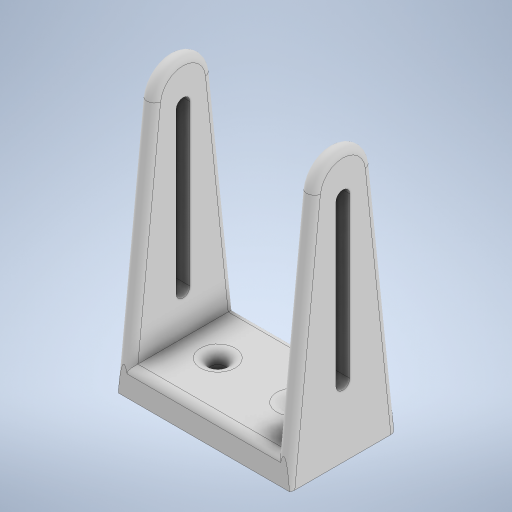
# Autodesk Inventor part: podstawa raspberry
Saved by Autodesk Inventor 2023 (Build 270158000, 158)
## iProperties
Created: 2023-04-25
Part Number: podstawa raspberry
Material: Ogólny
Document SubType Name: Modeling
Designer: janek
Density: 1 g/cm^3
Appearance: Domyślna
Author: janek
## iProperties of the stored document Zewnetrzny_stojak_Drukowanie 3D.ipt
Created: 2023-04-25
Part Number: Zewnetrzny_stojak_Drukowanie 3D
Material: Ogólny
Document SubType Name: Modeling
Designer: janek
Density: 1 g/cm^3
Appearance: Domyślna
Author: janek
Autodesk Inventor part; units mm, degrees
ref_plane "YZ Plane" through (0, 0, 0) normal (1, 0, 0) x (0, 1, 0)
ref_plane "XZ Plane" through (0, 0, 0) normal (0, 1, 0) x (-1, 0, 0)
ref_plane "XY Plane" through (0, 0, 0) normal (0, 0, 1) x (1, 0, 0)
sketch "Szkic1" plane through (0, 0, 0) normal (0, 1, 0) x (-1, 0, 0)
  line L0 (25.5952, -5.4437) -> (-24.4048, -5.4437)
  line L1 (-24.4048, -5.4437) -> (-24.4048, -35.4437)
  line L2 (-24.4048, -35.4437) -> (25.5952, -35.4437)
  line L3 (25.5952, -35.4437) -> (25.5952, -5.4437)
  point P0 (0, 0)
  point P1 (0.5952, -5.4437)
  point P2 (0.5952, -35.4437)
  dimension "d0" = 50
  dimension "d1" = 30
  constraints: 8 end point, 2 midpoint, 2 parallel, 1 horizontal, 1 perpendicular
  measures "d0" distance between parallel lines of L3 L1
  measures "d1" distance of point (0.595, -5.444) point (0.595, -35.444)
extrude "Wyciągnięcie proste1" add sketch "Szkic1" along normal blind 8
sketch "Szkic2" plane through (0, 8, 0) normal (0, 1, 0) x (1, 0, 0)
  line L0 (-25.5952, 35.4437) -> (-25.5952, 5.4437) projected
  line L1 (24.4048, 35.4437) -> (-25.5952, 35.4437) projected
  line L2 (-25.5952, 5.4437) -> (-21.5952, 5.4437)
  line L3 (-21.5952, 5.4437) -> (-21.5952, 35.4437)
  line L4 (-21.5952, 35.4437) -> (-25.5952, 35.4437)
  line L5 (-25.5952, 35.4437) -> (-25.5952, 5.4437)
  line L6 (-25.5952, 5.4437) -> (24.4048, 5.4437) projected
  line L7 (24.4048, 5.4437) -> (20.4048, 5.4437)
  line L8 (20.4048, 5.4437) -> (20.4048, 35.4437)
  line L9 (20.4048, 35.4437) -> (24.4048, 35.4437)
  line L10 (24.4048, 35.4437) -> (24.4048, 5.4437)
  point P0 (0, 0)
  dimension "d4" = 4
  dimension "d5" = 4
  constraints: 16 end point, 4 parallel, 2 horizontal, 2 perpendicular, 2 point on line
  measures "d4" distance between parallel lines of L8 L10
  measures "d5" distance between parallel lines of L0 L3
extrude "Wyciągnięcie proste2" add sketch "Szkic2" along normal blind 70 contours L1 L3 L2 L0 | L1 L10 L6 L8
chamfer "Faza1" distance 70 angle 6 1 edges at (-23.5952, 78, -5.4437) measured on face at (-7.5952, 2.6667, -5.4437)
chamfer "Faza2" distance 70 angle 6 1 edges at (22.4048, 78, -5.4437) measured on face at (-7.5952, 2.6667, -5.4437)
chamfer "Faza3" distance 70 angle 6 1 edges at (22.4048, 78, -35.4437) measured on face at (6.4048, 2.6667, -35.4437)
chamfer "Faza4" distance 70 angle 6 1 edges at (-23.5952, 78, -35.4437) measured on face at (6.4048, 2.6667, -35.4437)
sketch "Szkic3" plane through (-25.5952, 0, -35.4437) normal (-1, 0, 0) x (0, 0, 1)
  line L0 (13, 67.9596) -> (17, 67.9596)
  line L1 (17, 67.9596) -> (17, 17.9596)
  line L2 (17, 17.9596) -> (13, 17.9596)
  line L3 (13, 17.9596) -> (13, 67.9596)
  line L4 (7.3573, 78) -> (22.6427, 78) projected
  point P0 (35.4437, 0)
  point P1 (15, 67.9596)
  point P2 (15, 78)
  point P3 (15, 78)
  point P4 (15, 17.9596)
  dimension "d20" = 4
  dimension "d21" = 10.0404
  dimension "d22" = 50
  constraints: 8 end point, 4 midpoint, 2 parallel, 1 horizontal, 1 perpendicular, 1 vertical alignment
  measures "d20" distance between parallel lines of L1 L3
  measures "d21" distance of point (15, 78) point (15, 67.96)
  measures "d22" distance of point (15, 67.96) point (15, 17.96)
extrude "Wyciągnięcie proste3" cut sketch "Szkic3" against normal blind 70
sketch "Szkic4" plane through (0, 8, 0) normal (0, 1, 0) x (1, 0, 0)
  circle A0 centre (10.4048, 20.4437) radius 2
  circle A1 centre (-11.5952, 20.4437) radius 2
  line L0 (20.4048, 28.0864) -> (20.4048, 12.801) projected
  line L1 (-21.5952, 12.801) -> (-21.5952, 28.0864) projected
  point P0 (0, 0)
  point P1 (20.4048, 20.4437)
  point P2 (-21.5952, 20.4437)
  point P3 (-21.5952, 20.4437)
  point P4 (20.4048, 20.4437)
  dimension "d25" = 4
  dimension "d26" = 4
  dimension "d27" = 10
  dimension "d28" = 10
  constraints: 4 midpoint, 2 centre point, 2 horizontal alignment
  measures "d25" diameter of A1
  measures "d26" diameter of A0
  measures "d27" distance of A1.centre point (-21.595, 20.444)
  measures "d28" distance of point (20.405, 20.444) A0.centre
extrude "Wyciągnięcie proste4" cut sketch "Szkic4" against normal blind 70
fillet "Zaokrąglenie1" radius 3 2 edges at (-13.5952, 8, -20.4437) (8.4048, 8, -20.4437)
fillet "Zaokrąglenie2" radius 2 8 edges at (-23.5952, 67.9596, -22.4437) (-23.5952, 67.9596, -18.4437) (-23.5952, 17.9596, -22.4437) (-23.5952, 17.9596, -18.4437) (22.4048, 17.9596, -18.4437) (22.4048, 17.9596, -22.4437) (22.4048, 67.9596, -18.4437) (22.4048, 67.9596, -22.4437)
fillet "Zaokrąglenie3" radius 8.5 4 edges at (22.4048, 78, -12.801) (22.4048, 78, -28.0864) (-23.5952, 78, -12.801) (-23.5952, 78, -28.0864)
fillet "Zaokrąglenie4" radius 2 14 edges at (24.4048, 77.9065, -20.4437) (24.4048, 39.1479, -8.7175) (24.4048, 39.1479, -32.1699) (20.4048, 77.9065, -20.4437) (20.4048, 39.1479, -8.7175) (20.4048, 39.1479, -32.1699) (-21.5952, 77.9065, -20.4437) (-21.5952, 39.1479, -8.7175) (-21.5952, 39.1479, -32.1699) (-25.5952, 77.9065, -20.4437) (-25.5952, 39.1479, -8.7175) (-25.5952, 39.1479, -32.1699) (-0.5952, 8, -35.4437) (-0.5952, 8, -5.4437)
